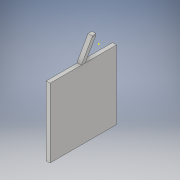
# Autodesk Inventor part: ClawPaddle
Saved by Autodesk Inventor 2017 (Build 210142000, 142)
## iProperties
Created: 2017-09-23
Part Number: ClawPaddle
Material: Generic
Document SubType Name: Modeling
Designer: User
Density: 1 g/cm^3
Appearance: Default
Author: User
Autodesk Inventor part; units mm, degrees
ref_plane "YZ Plane" through (0, 0, 0) normal (1, 0, 0) x (0, 1, 0)
ref_plane "XZ Plane" through (0, 0, 0) normal (0, 1, 0) x (-1, 0, 0)
ref_plane "XY Plane" through (0, 0, 0) normal (0, 0, 1) x (1, 0, 0)
sketch "Sketch1" plane through (0, 0, 0) normal (1, 0, 0) x (0, 1, 0)
  line L0 (0, 0) -> (56.134, 0)
  line L1 (56.134, 0) -> (56.134, -3.175)
  line L2 (56.134, -3.175) -> (0, -3.175)
  line L3 (0, -3.175) -> (0, 0)
  dimension "d0" = 56.134
  dimension "d1" = 3.175
  constraints: 8 end point, 2 horizontal, 1 perpendicular, 1 vertical
  measures "d0" distance of L0.start L0.end
  measures "d1" distance of L0.end L1.end
extrude "Extrusion1" add sketch "Sketch1" along normal blind 25.4
sketch "Sketch2" plane through (0, 56.134, 0) normal (0, 1, 0) x (1, 0, 0)
  line L0 (0, 3.175) -> (25.4, 3.175) projected
  line L1 (11.1125, 3.175) -> (11.1125, 0)
  line L2 (14.2875, 0) -> (14.2875, 3.175)
  line L3 (11.1125, 3.175) -> (14.2875, 3.175)
  line L4 (14.2875, 0) -> (11.1125, 0)
  line L5 (0, 3.175) -> (25.4, 3.175) projected
  line L6 (0, 0) -> (0, 3.175) projected
  line L7 (0, 0) -> (25.4, 0) projected
  line L8 (25.4, 3.175) -> (25.4, 0) projected
  line L9 (0, 3.175) -> (25.4, 3.175) projected
  line L10 (14.2875, 0) -> (11.1125, 0)
  constraints: 10 end point, 2 collinear, 2 point on line, 1 parallel, 1 perpendicular
sketch "Sketch3" plane through (0, 0, 0) normal (0, 0, 1) x (1, 0, 0)
  line L0 (14.2875, 56.134) -> (11.1125, 57.2894)
  line L1 (11.1125, 57.2894) -> (11.1125, 56.134)
  line L2 (0, 56.134) -> (25.4, 56.134) projected
  point P0 (0, 0)
  constraints: 4 end point, 1 perpendicular
extrude "Extrusion2" add sketch "Sketch3" against normal blind 3.175
sketch "Sketch4" plane through (14.2875, 56.134, 0) normal (0.341963, 0.9397134, 0) x (0.9397134, -0.341963, 0)
  line L0 (0, 3.175) -> (0, 0) projected
  line L1 (-3.3787, 0) -> (-3.3787, 3.175) projected
  line L2 (0, 3.175) -> (-3.3787, 3.175)
  line L3 (-3.3787, 3.175) -> (-3.3787, 0)
  line L4 (-3.3787, 0) -> (0, 0)
  line L5 (0, 0) -> (0, 3.175)
  point P0 (5.7696, 0)
  constraints: 8 end point, 2 parallel, 1 horizontal, 1 perpendicular
extrude "Extrusion3" add sketch "Sketch4" along normal blind 25.4
sketch "Sketch5" plane through (22.9734, 80.0027, 0) normal (0.341963, 0.9397134, 0) x (0.9397134, -0.341963, 0)
  point P0 (5.7696, 0)
sketch "Sketch6" plane through (0, 0, -3.175) normal (0, 0, -1) x (-1, 0, 0)
  line L0 (-19.7984, 81.1581) -> (-22.9734, 80.0027) projected
  line L1 (-19.7984, 81.1581) -> (-22.9734, 81.1581)
  line L2 (-22.9734, 81.1581) -> (-22.9734, 80.0027)
  point P0 (0, 0)
  constraints: 4 end point, 1 horizontal, 1 perpendicular
extrude "Extrusion4" add sketch "Sketch6" against normal blind 3.175
sketch "Sketch7" plane through (0, 0, 0) normal (0, 0, 1) x (1, 0, 0)
  line L0 (0, 56.134) -> (11.1125, 56.134) projected
  line L1 (11.1125, 56.134) -> (11.1125, 0)
  line L2 (0, 0) -> (25.4, 0) projected
  line L3 (11.1125, 0) -> (0, 0)
  line L4 (0, 0) -> (0, 56.134) projected
  line L5 (0, 0) -> (0, 56.134)
  line L6 (14.2875, 56.134) -> (25.4, 56.134) projected
  line L7 (14.2875, 56.134) -> (14.2875, 0)
  line L8 (25.4, 56.134) -> (25.4, 0) projected
  line L9 (25.4, 0) -> (25.4, 56.134)
  constraints: 10 end point, 2 perpendicular, 2 vertical, 1 collinear, 1 point on line
extrude "Extrusion5" cut sketch "Sketch7" against normal blind 25.4
sketch "Sketch8" plane through (11.1125, 0, 0) normal (0, 0, 1) x (1, 0, 0)
  line L0 (3.175, 56.134) -> (11.8609, 80.0027) projected
  line L1 (3.175, 56.134) -> (0, 56.134)
  line L2 (0, 0) -> (0, 57.2894) projected
  line L3 (0, 0) -> (3.175, 0) projected
  line L4 (3.175, 0) -> (0, 0)
  line L5 (3.175, 56.134) -> (3.175, 0)
  point P0 (-11.1125, 0)
  constraints: 6 end point, 1 collinear, 1 horizontal, 1 perpendicular, 1 point on line
extrude "Extrusion6" add sketch "Sketch8" along normal blind 25.4
sketch "Sketch9" plane through (11.1125, 0, -3.175) normal (0, 0, -1) x (-1, 0, 0)
  line L0 (0, 0) -> (-3.175, 0) projected
  line L1 (-3.175, 56.134) -> (-3.175, 0) projected
  line L2 (0, 0) -> (-3.175, 0)
  line L3 (-3.175, 0) -> (-3.175, 56.134)
  line L4 (-3.175, 56.134) -> (0, 56.134)
  line L5 (0, 56.134) -> (0, 0)
  point P0 (11.1125, 0)
  constraints: 8 end point, 2 parallel, 1 horizontal, 1 perpendicular
extrude "Extrusion7" add sketch "Sketch9" along normal blind 25.4
body "Solid1"
